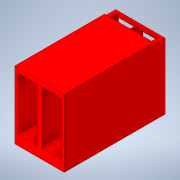
# Autodesk Inventor part: 10_cube_active_solution_chamber_90mm_with_top_DOUBLE
Saved by Autodesk Inventor 2022 (Build 260153000, 153)
## iProperties
Created: 2017-06-20
Part Number: 10_cube_active_solution_chamber_90mm_with_top_DOUBLE
Material: Generisch
Document SubType Name: Modeling
Designer: diederichbenedict
Density: 1 g/cm^3
Appearance: Weiß
Mass: 7.87446 g
Surface Area: 71.4468 cm^2
Volume: 7.87446 cm^3
d_part: 50,000 mm
d_o: 40,000 mm
d_i: 40,000 mm
Author: diederichbenedict
Autodesk Inventor part; units mm, degrees
ref_plane "YZ Plane" through (0, 0, 0) normal (1, 0, 0) x (0, 1, 0)
ref_plane "XZ Plane" through (0, 0, 0) normal (0, 1, 0) x (-1, 0, 0)
ref_plane "XY Plane" through (0, 0, 0) normal (0, 0, 1) x (1, 0, 0)
sketch "Skizze1" plane through (0, 0, 0) normal (0, 0, 1) x (1, 0, 0)
  line L0 (-15, 15) -> (15, -15) construction
  line L1 (15, 15) -> (-15, -15) construction
  line L2 (-22, 45) -> (22, 45)
  line L3 (22, 45) -> (22, -45)
  line L4 (22, -45) -> (-22, -45)
  line L5 (-22, -45) -> (-22, 45)
  line L6 (-22, 45) -> (22, -45) construction
  line L7 (22, 45) -> (-22, -45) construction
  line L8 (11.5, 19.9186) -> (11.5, -19.9186) construction
  line L9 (20, -20) -> (-20, -20) construction
  line L10 (-20, 20) -> (20, 20) construction
  line L11 (20, 20) -> (20, -20) construction
  line L12 (20, -20) -> (-20, 20) construction
  line L13 (-20, -20) -> (20, 20) construction
  line L14 (17.5, 17.5) -> (-17.5, -17.5) construction
  line L15 (-17.5, 17.5) -> (17.5, -17.5) construction
  point P0 (0, 0)
  point P1 (0, 0)
  dimension "d2" = 44
  dimension "d3" = 90
  constraints: 32 end point, 8 midpoint, 4 coincident, 3 parallel, 2 horizontal, 1 perpendicular, 2 other
  measures "d2" distance of L3.end L4.end
  measures "d3" distance of L2.end L3.end
extrude "Extrusion1" add sketch "Skizze1" along normal blind 9
ref_plane "Arbeitsebene1" through (-22, -40, 0) normal (0, -1, 0) x (1, 0, 0)
sketch "Skizze5" plane through (-22, -40, 0) normal (0, -1, 0) x (1, 0, 0)
  line L0 (44, 9) -> (0, 9) projected
  line L1 (0, 9) -> (44, 9) projected
  arc A0 (7.65, -12.2861) -> (5, -9.6361) centre (5, -12.2861) ccw
  line L2 (7.65, -14.7934) -> (7.65, -19.2214)
  line L3 (7.65, -19.2214) -> (5, -19.2214)
  line L4 (5, -9.6361) -> (5, -19.2214)
  line L5 (0, 0) -> (0, 9) projected
  arc A1 (7.1796, -13.7934) -> (5, -9.6361) centre (5, -12.2861) ccw
  line L6 (7.1796, -13.7934) -> (7.1796, -14.7934) construction
  line L7 (7.1796, -13.7934) -> (8.1796, -13.7934) construction
  line L8 (7.1796, -14.7934) -> (7.65, -14.7934) construction
  line L9 (7.1796, -13.7934) -> (7.65, -14.7934)
  line L10 (-2.9393, -5.484) -> (12.0607, -5.484)
  arc A2 (5, -1.3318) -> (7.65, 1.3182) centre (5, 1.3182) ccw
  line L11 (7.65, 3.8254) -> (7.65, 8.2534)
  line L12 (7.65, 8.2534) -> (5, 8.2534)
  line L13 (5, -1.3318) -> (5, 8.2534)
  arc A3 (5, -1.3318) -> (7.1796, 2.8254) centre (5, 1.3182) ccw
  line L14 (7.1796, 2.8254) -> (7.1796, 3.8254) construction
  line L15 (7.1796, 2.8254) -> (8.1796, 2.8254) construction
  line L16 (7.1796, 3.8254) -> (7.65, 3.8254) construction
  line L17 (7.1796, 2.8254) -> (7.65, 3.8254)
  line L18 (0, 0) -> (44, 0) projected
  line L19 (0, 0) -> (0, 9) projected
  line L20 (44, 9) -> (0, 9) projected
  line L21 (44, 0) -> (44, 9) projected
  point P0 (22, 0)
  point P1 (10, 8)
  point P2 (40, 8)
  point P3 (6.6949, -37.8745)
  point P4 (5, -8.3675)
  point P5 (5, -2.6005)
  dimension "d85" = 5.3
  dimension "d86" = 2.65
  dimension "d87" = 9.5853
  dimension "d88" = 6.9353
  dimension "d89" = 5
  dimension "d91" = 1
  dimension "d92" = 90
  constraints: 30 end point, 17 symmetric about line, 12 coincident, 12 point on circle, 4 centre point, 4 point on line, 2 horizontal, 2 perpendicular, 2 vertical, 1 concentric, 6 other
  measures "d85" diameter of A0
  measures "d86" distance between parallel lines of L2 L4
  measures "d87" distance of L4.start L3.end
  measures "d88" distance from line of A0.centre L3
  measures "d89" distance between parallel lines of L5 L4
  measures "d91" distance of L6.start L6.end
  measures "d92" angle of L6 L7
revolve "Umdrehung1" cut sketch "Skizze5" angle 360 about axis through (-17, -40, -9.6361) along (0, 0, -1) contours L18 L13 L12 L11 L17 A3 A2 | A2 L13 L18 | A1 L9 L2 L3 L4 A0
mirror "Spiegeln7" about plane through (0, 0, 0) normal (0, 1, 0) of "Umdrehung1"
sketch "Skizze18" plane through (0, 0, 0) normal (0, 0, -1) x (-1, 0, 0)
  circle A0 centre (0, 0) radius 17.5
  constraints: 1 centre point, 1 coincident
pattern_circular "Runde Anordnung3" count 4 over 360 about axis through (0, 0, 0) along (0, 0, 1) of "Umdrehung1", "Spiegeln7"
sketch "Skizze24" plane through (0, 0, 9) normal (0, 0, 1) x (1, 0, 0)
  line L0 (-22, -45) -> (-22, -43)
  line L1 (-18.5, 43) -> (-0.75, 43)
  line L2 (18.5, -43) -> (0.75, -43)
  line L3 (-18.5, -43) -> (-18.5, 43)
  line L4 (-18.5, 43) -> (-0.75, 1.7432) construction
  line L5 (18.5, 43) -> (0.75, 1.7432) construction
  line L6 (0.75, 43) -> (0.75, 1.7432)
  line L7 (-0.75, -43) -> (-0.75, -1.7432)
  line L8 (0.75, 43) -> (18.5, 43)
  line L9 (-0.75, 1.7432) -> (-0.75, 43)
  line L10 (0.75, 1.7432) -> (0.75, -0.3125)
  line L11 (0.75, -0.3125) -> (0.75, -43)
  line L12 (-0.75, -43) -> (-18.5, -43)
  line L13 (-0.75, -1.7432) -> (-0.75, 1.7432)
  line L14 (18.5, -43) -> (22, -45) construction
  line L15 (0.75, 1.7432) -> (-0.75, -1.7432) construction
  line L16 (18.5, 43) -> (0.75, 1.7432) construction
  line L17 (0.75, 1.7432) -> (-0.75, -1.7432) construction
  line L18 (-22, -43) -> (-22, 43)
  line L19 (-22, 43) -> (-22, 45)
  line L20 (0.75, -0.3125) -> (18.5, -43) construction
  line L21 (18.5, -43) -> (18.5, 43)
  line L22 (0.75, -0.3125) -> (18.5, -43) construction
  line L23 (-22, -45) -> (-18.5, -45)
  line L24 (-18.5, -45) -> (-0.75, -45)
  line L25 (-18.5, -43) -> (-22, -45) construction
  line L26 (-0.75, -45) -> (0.75, -45)
  line L27 (22, -43) -> (22, -45)
  line L28 (18.5, -45) -> (22, -45)
  line L29 (22, 43) -> (22, -43)
  line L30 (0.75, -45) -> (18.5, -45)
  line L31 (-18.5, 43) -> (-0.75, 1.7432) construction
  line L32 (-0.75, -1.7432) -> (-18.5, -43) construction
  line L33 (-0.75, -1.7432) -> (-18.5, -43) construction
  line L34 (-0.75, 1.7432) -> (0, 0) construction
  line L35 (-0.75, 1.7432) -> (0, 0) construction
  line L36 (0, 0) -> (0.75, -0.3125) construction
  line L37 (0, 0) -> (0.75, -0.3125) construction
  line L38 (22, 45) -> (-22, 45) projected
  line L39 (22, 45) -> (20, 45)
  line L40 (-20, 45) -> (-22, 45)
  line L41 (20, 45) -> (18.5, 43) construction
  line L42 (20, 45) -> (19.3605, 45)
  line L43 (22, 45) -> (22, 43)
  line L44 (19.3605, 45) -> (18.5, 45)
  line L45 (18.5, 45) -> (-0.75, 45)
  line L46 (-18.5, 45) -> (-18.0915, 45)
  line L47 (-0.75, 45) -> (-18.5, 45)
  line L48 (-20, 45) -> (-18.5, 43) construction
  line L49 (-18.0915, 45) -> (-20, 45)
  point P0 (0, 41.625)
  point P1 (0, 41.625)
  point P2 (0, 41.625)
  point P3 (0, 45)
  point P4 (20, -43)
  dimension "d252" = 1.5
  dimension "d253" = 17.75
  dimension "d254" = 17.75
  dimension "d260" = 2
  dimension "d261" = 2
  dimension "d262" = 2
  dimension "d263" = 2
  constraints: 98 end point, 19 point on line, 16 parallel, 8 collinear, 7 horizontal, 2 midpoint, 1 coincident, 1 vertical, 1 vertical alignment
  measures "d252" distance between parallel lines of L7 L6
  measures "d253" distance between parallel lines of L7 L3
  measures "d254" distance between parallel lines of L21 L11
  measures "d260" distance between parallel lines of L12 L24
  measures "d261" distance between parallel lines of L2 L30
  measures "d262" distance between parallel lines of L1 L38
  measures "d263" distance between parallel lines of L38 L8
extrude "Extrusion12" add sketch "Skizze24" along normal blind 50
sketch "Skizze25" plane through (-22, -45, 0) normal (0, -1, 0) x (1, 0, 0)
  line L0 (0, 0) -> (0, 59) projected
  line L1 (2.5, 56) -> (2.5, 9)
  line L2 (2.5, 9) -> (19.75, 9)
  line L3 (19.75, 9) -> (19.75, 56)
  line L4 (19.75, 56) -> (2.5, 56)
  line L5 (44, 0) -> (44, 59) projected
  line L6 (44, 0) -> (0, 0) projected
  line L7 (0, 59) -> (44, 59) projected
  point P0 (22, 0)
  point P1 (12.5, 20)
  point P2 (20, 46)
  point P3 (20, 49)
  dimension "d249" = 2.5
  dimension "d251" = 9
  dimension "d255" = 17.25
  dimension "d259" = 3
  constraints: 8 end point, 2 parallel, 1 perpendicular, 1 vertical, 1 vertical alignment
  measures "d249" distance between parallel lines of L0 L1
  measures "d251" distance between parallel lines of L6 L2
  measures "d255" distance between parallel lines of L3 L1
  measures "d259" distance between parallel lines of L7 L4
extrude "Extrusion13" cut sketch "Skizze25" against normal up to surface (90 mm away) contours L4 L3 L2 L1
mirror "Mirror8" about plane through (0, 0, 0) normal (1, 0, 0) of "Extrusion13"
sketch "Sketch26" plane through (-22, -45, 0) normal (0, -1, 0) x (1, 0, 0)
  line L0 (0, 0) -> (0, 59) projected
  line L1 (0, 59) -> (44, 59) projected
  line L2 (0, 59) -> (44, 59)
  line L3 (44, 59) -> (44, 60.5)
  line L4 (44, 60.5) -> (0, 60.5)
  line L5 (0, 60.5) -> (0, 59)
  point P0 (22, 0)
  dimension "d256" = 1.5
  constraints: 8 end point, 2 parallel, 1 horizontal, 1 perpendicular
  measures "d256" distance between parallel lines of L1 L4
extrude "Extrusion14" add sketch "Sketch26" against normal blind 80
ref_plane "Arbeitsebene8" through (0, 0, -11.3) normal (0, 0, -1) x (0, -1, 0)
ref_plane "Arbeitsebene9" through (0, 0, -11.3) normal (0, 0, -1) x (1, 0, 0)
ref_plane "Arbeitsebene10" through (0, 0, -11.3) normal (0, 0, -1) x (0, 1, 0)
ref_plane "Arbeitsebene14" through (25, 0, -11.3) normal (0, 0, 1) x (1, 0, 0)
equation "\"d_i\" = 40"
equation "\"d_o\" = 40"
equation "\"d_part\" = 50"
equation "\"d6\" = 0"
equation "\"d7\" = 0"
equation "\"d8\" = 0"
equation "\"d9\" = 0"
equation "\"d13\" = 0"
equation "\"d14\" = 0"
equation "\"d20\" = 0"
equation "\"d21\" = 0"
equation "\"d22\" = 0"
equation "\"d23\" = 0"
equation "\"d24\" = 0"
equation "\"d25\" = 3"
equation "\"d26\" = 0"
equation "\"d27\" = 0"
equation "\"d28\" = 0"
equation "\"d29\" = 0"
equation "\"d30\" = 0"
equation "\"d31\" = 0"
equation "\"d32\" = 0"
equation "\"d33\" = 0"
equation "\"d34\" = 0"
equation "\"d46\" = 0"
equation "\"d47\" = 0"
equation "\"d48\" = 0"
equation "\"d50\" = 0"
equation "\"d51\" = 0"
equation "\"d52\" = 0"
equation "\"d53\" = 0"
equation "\"d54\" = 0"
equation "\"d55\" = 0"
equation "\"d56\" = 0"
equation "\"d57\" = 0"
equation "\"d58\" = 0"
equation "\"d59\" = 0"
